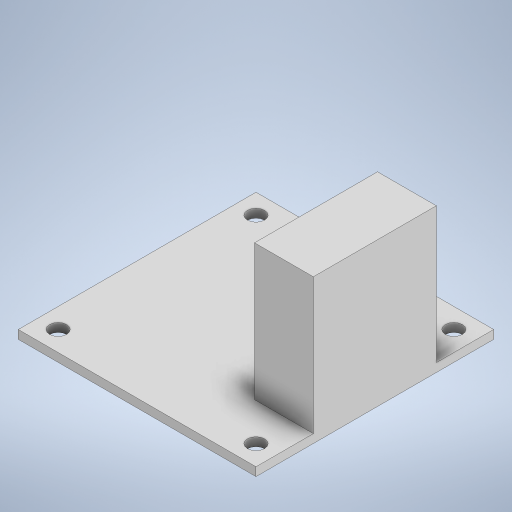
# Autodesk Inventor part: l298n
Saved by Autodesk Inventor 2024 (Build 280153000, 153)
## iProperties
Created: 2024-04-10
Part Number: l298n
Material: 一般
Document SubType Name: Modeling
Designer: rumse
Density: 1 g/cm^3
Appearance: 預設
Author: rumse
Autodesk Inventor part; units mm, degrees
ref_plane "YZ Plane" through (0, 0, 0) normal (1, 0, 0) x (0, 1, 0)
ref_plane "XZ Plane" through (0, 0, 0) normal (0, 1, 0) x (-1, 0, 0)
ref_plane "XY Plane" through (0, 0, 0) normal (0, 0, 1) x (1, 0, 0)
sketch "草圖1" plane through (0, 0, 0) normal (0, 1, 0) x (-1, 0, 0)
  line L0 (0, 0) -> (44.45, 0)
  line L1 (44.45, 0) -> (44.45, -44.45)
  line L2 (44.45, -44.45) -> (0, -44.45)
  line L3 (0, -44.45) -> (0, 0)
  line L4 (3.725, -3.725) -> (40.725, -3.725)
  line L5 (40.725, -3.725) -> (40.725, -40.725)
  line L6 (40.725, -40.725) -> (3.725, -40.725)
  line L7 (3.725, -40.725) -> (3.725, -3.725)
  circle A0 centre (40.725, -3.725) radius 1.6
  circle A1 centre (40.725, -40.725) radius 1.6
  circle A2 centre (3.725, -3.725) radius 1.6
  circle A3 centre (3.725, -40.725) radius 1.6
  line L8 (11, -33.725) -> (0, -33.725)
  line L9 (0, -33.725) -> (0, -10.725)
  line L10 (0, -10.725) -> (11, -10.725)
  line L11 (11, -10.725) -> (11, -33.725)
  point P0 (0, -33.725)
  dimension "d0" = 44.45
  dimension "d1" = 44.45
  dimension "d2" = 37
  dimension "d3" = 37
  dimension "d4" = 3.725
  dimension "d5" = 3.725
  dimension "d6" = 3.2
  dimension "d7" = 3.2
  dimension "d8" = 3.2
  dimension "d9" = 3.2
  dimension "d14" = 23
  dimension "d15" = 11
  dimension "d16" = 10.725
  constraints: 24 end point, 6 parallel, 4 centre point, 4 coincident, 3 horizontal, 3 perpendicular, 1 point on line
  measures "d0" distance of L0.end L1.end
  measures "d1" distance of L1.end L2.end
  measures "d2" distance of L4.end L5.end
  measures "d3" distance of L5.end L6.end
  measures "d4" horizontal distance of L0.start L4.start
  measures "d5" horizontal distance of L0.start L4.start
  measures "d6" diameter of A0
  measures "d7" diameter of A1
  measures "d8" diameter of A2
  measures "d9" diameter of A3
  measures "d14" distance of L10.end L8.start
  measures "d15" distance of L9.end L10.end
  measures "d16" distance of L0.start L9.end
extrude "擠出1" add sketch "草圖1" along normal blind 27 contours L10 L7 L8 L3 | L10 L11 L8 L7
extrude "擠出2" cut sketch "草圖1" along normal blind 27 contours A2 L4 L7 | L7 L4 A2 | A3 L6 L7 | L7 L6 A3 | A0 L5 L4 | L4 L5 A0 | A1 L5 L6 | L6 L5 A1
extrude "擠出3" add sketch "草圖1" along normal blind 1.6 contours L0 L1 L2 L3 L8 L7 A3 L6 A1 L5 A0 L4 A2 L10 | L7 A2 L4 A0 L5 A1 L6 A3 L8 L11 L10
